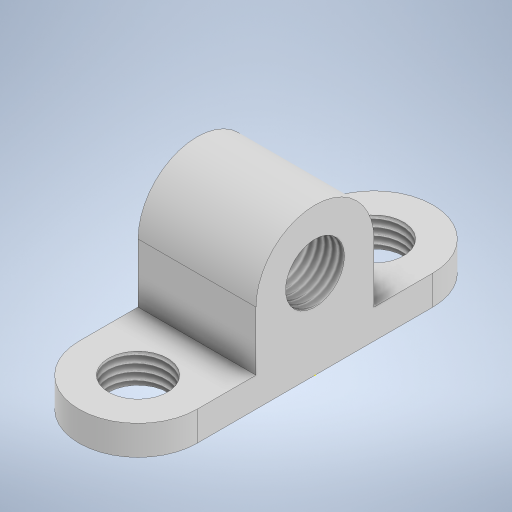
# Autodesk Inventor part: TAREA #1-1021920
Saved by Autodesk Inventor 2024 (Build 280153000, 153)
## iProperties
Created: 2024-01-23
Part Number: TAREA #1-1021920
Material: Generic
Document SubType Name: Modeling
Designer: JavierJ
Density: 1 g/cm^3
Appearance: Default
Author: JavierJ
Autodesk Inventor part; units mm, degrees
ref_plane "YZ Plane" through (0, 0, 0) normal (1, 0, 0) x (0, 1, 0)
ref_plane "XZ Plane" through (0, 0, 0) normal (0, 1, 0) x (-1, 0, 0)
ref_plane "XY Plane" through (0, 0, 0) normal (0, 0, 1) x (1, 0, 0)
sketch "Sketch1" plane through (0, 0, 0) normal (0, 0, 1) x (1, 0, 0)
  point P0 (0, 0)
sketch "Sketch2" plane through (0, 0, 0) normal (0, 1, 0) x (-1, 0, 0)
  line L0 (-20, -20) -> (-20, 20)
  line L1 (20, 20) -> (20, -20)
  line L2 (20, -20) -> (-20, 20) construction
  line L3 (-20, -20) -> (20, 20) construction
  arc A0 (20, 40) -> (-20, 40) centre (0, 40) ccw
  circle A1 centre (0, 40) radius 10
  arc A2 (-20, -40) -> (20, -40) centre (0, -40) ccw
  circle A3 centre (0, -40) radius 10
  line L4 (20, 20) -> (20, 40)
  line L5 (20, -20) -> (20, -40)
  line L6 (-20, 40) -> (-20, 20)
  line L7 (-20, -20) -> (-20, -40)
  point P0 (0, 0)
  constraints: 16 end point, 4 centre point, 4 point on circle, 2 coincident, 2 midpoint, 2 vertical, 1 parallel, 1 tangent
extrude "Extrusion1" add sketch "Sketch2" along normal blind 10
sketch "Sketch3" plane through (20, 0, 40) normal (1, 0, 0) x (0, 0, -1)
  line L0 (80, 10) -> (0, 10) construction
  line L1 (40, 10) -> (40, 30) construction
  circle A0 centre (40, 30) radius 10
  arc A1 (60, 30) -> (20, 30) centre (40, 30) ccw
  line L2 (20, 30) -> (20, 10)
  line L3 (60, 30) -> (60, 10)
  line L4 (20, 10) -> (60, 10)
  point P0 (40, 0)
  constraints: 8 end point, 3 vertical, 2 centre point, 2 coincident, 2 point on circle, 2 tangent, 1 collinear, 1 midpoint
extrude "Extrusion2" add sketch "Sketch3" against normal blind 40
thread "Thread1" size "M20x2.5" class "6H" standard "ANSI Metric M Profile" full length
thread "Thread2" size "M20x2.5" class "6H" standard "ANSI Metric M Profile" full length
thread "Thread3" size "M20x2.5" class "6H" standard "ANSI Metric M Profile" full length
sketch "Sketch4" plane through (20, 0, 40) normal (1, 0, 0) x (0, 0, -1)
  point P0 (40, 0)
body "Solid1"
